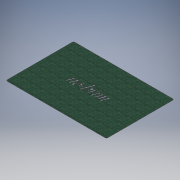
# Autodesk Inventor part: Lamiera logo no-brim
Saved by Autodesk Inventor 2018 (Build 220112000, 112)
## iProperties
Created: 2020-06-01
Part Number: Lamiera logo no-brim
Material: Generico
Document SubType Name: Lamiera
Designer: Francesco
Density: 1 g/cm^3
Sheet Metal Rule: Default_mm
Appearance: Verde - Lucido
Author: Francesco
Autodesk Inventor part; units mm, degrees
ref_plane "YZ Plane" through (0, 0, 0) normal (1, 0, 0) x (0, 1, 0)
ref_plane "XZ Plane" through (0, 0, 0) normal (0, 1, 0) x (-1, 0, 0)
ref_plane "XY Plane" through (0, 0, 0) normal (0, 0, 1) x (1, 0, 0)
sketch "Schizzo1" plane through (0, 0, 0) normal (0, 0, 1) x (1, 0, 0)
  line L0 (-335, 225.25) -> (335, 225.25)
  line L1 (335, 225.25) -> (335, -225.25)
  line L2 (335, -225.25) -> (-335, -225.25)
  line L3 (-335, -225.25) -> (-335, 225.25)
  line L4 (-335, 225.25) -> (335, -225.25) construction
  line L5 (335, 225.25) -> (-335, -225.25) construction
  point P0 (0, 0)
  dimension "d0" = 670
  dimension "d1" = 450.5
  measures "d0" distance of L1.end L2.end
  measures "d1" distance of L0.end L1.end
extrude "Piano1" add sketch "Schizzo1" along normal blind 1
fillet "Arrotondamento angolo1" radius 10 4 edges at (335, 225.25, 0.5) (-335, 225.25, 0.5) (335, -225.25, 0.5) (-335, -225.25, 0.5)
sketch "Schizzo2" plane through (0, 0, 1) normal (0, 0, 1) x (1, 0, 0)
  line L0 (-157.4575, 51.7567) -> (134.7822, 51.7567) construction
  line L1 (134.7822, 51.7567) -> (134.7822, -31.7703) construction
  line L2 (134.7822, -31.7703) -> (-157.4575, -31.7703) construction
  line L3 (-157.4575, -31.7703) -> (-157.4575, 51.7567) construction
  line L4 (-101.4621, -20.1147) -> (-100.5991, -21.6417)
  spline S0 degree 2 poles (-100.5991, -21.6417) (-107.3044, -26.4218) (-116.4663, -28.3471) knots 0 0 0 1 1 1
  spline S1 degree 2 poles (-116.4663, -28.3471) (-115.2713, -19.1189) (-105.5783, -0.3305) knots 0 0 0 1 1 1
  line L5 (-105.5783, -0.3305) -> (-101.9932, 6.5741)
  spline S2 degree 2 poles (-101.9932, 6.5741) (-100.1343, 10.1592) (-100.1343, 11.155) knots 0 0 0 1 1 1
  spline S3 degree 2 poles (-100.1343, 11.155) (-100.1343, 12.682) (-101.3293, 12.682) knots 0 0 0 1 1 1
  spline S4 degree 2 poles (-101.3293, 12.682) (-103.1219, 12.682) (-112.7484, 4.848) (-117.3293, -0.2641) knots 0 0 0 1 2 2 2
  spline S5 degree 2 poles (-117.3293, -0.2641) (-126.8231, -10.8865) (-133.263, -25.7579) knots 0 0 0 1 1 1
  spline S6 degree 2 poles (-133.263, -25.7579) (-135.8522, -26.3554) (-140.6322, -28.4135) knots 0 0 0 1 1 1
  spline S7 degree 2 poles (-140.6322, -28.4135) (-135.5202, -17.9238) (-125.097, 8.2338) (-125.097, 10.6239) knots 0 0 0 1 2 2 2
  spline S8 degree 2 poles (-125.097, 10.6239) (-125.097, 12.6156) (-126.6903, 12.6156) knots 0 0 0 1 1 1
  spline S9 degree 2 poles (-126.6903, 12.6156) (-127.5534, 12.6156) (-130.3418, 11.7525) knots 0 0 0 1 1 1
  spline S10 degree 2 poles (-130.3418, 11.7525) (-130.541, 11.6861) (-130.9393, 11.6197) knots 0 0 0 1 1 1
  line L6 (-130.9393, 11.6197) -> (-131.2713, 13.3459)
  spline S11 degree 2 poles (-131.2713, 13.3459) (-123.4372, 15.6031) (-117.1302, 18.3915) knots 0 0 0 1 1 1
  line L7 (-117.1302, 18.3915) -> (-116.4663, 18.7235)
  spline S12 degree 2 poles (-116.4663, 18.7235) (-116.3335, 17.9932) (-116.3335, 17.7276) knots 0 0 0 1 1 1
  spline S13 degree 2 poles (-116.3335, 17.7276) (-116.3335, 12.7484) (-123.6364, -3.3844) knots 0 0 0 1 1 1
  line L8 (-123.6364, -3.3844) -> (-124.4331, -5.0442)
  line L9 (-124.4331, -5.0442) -> (-123.4372, -3.9819)
  spline S14 degree 2 poles (-123.4372, -3.9819) (-114.3418, 6.4413) (-98.8729, 18.4579) (-94.4912, 18.4579) knots 0 0 0 1 2 2 2
  spline S15 degree 2 poles (-94.4912, 18.4579) (-91.7692, 18.4579) (-91.7692, 15.6695) knots 0 0 0 1 1 1
  spline S16 degree 2 poles (-91.7692, 15.6695) (-91.7692, 12.7484) (-99.0721, -1.4591) knots 0 0 0 1 1 1
  spline S17 degree 2 poles (-99.0721, -1.4591) (-107.8356, -18.4549) (-107.8356, -20.5794) knots 0 0 0 1 1 1
  spline S18 degree 2 poles (-107.8356, -20.5794) (-107.8356, -22.1728) (-106.3086, -22.1728) knots 0 0 0 1 1 1
  spline S19 degree 2 poles (-106.3086, -22.1728) (-104.6488, -22.1728) (-101.7941, -20.3803) knots 0 0 0 1 1 1
  line L10 (-101.7941, -20.3803) -> (-101.4621, -20.1147)
  spline S20 degree 2 poles (-53.7941, 12.9475) (-56.7152, 13.2131) (-58.7069, 13.2131) knots 0 0 0 1 1 1
  spline S21 degree 2 poles (-58.7069, 13.2131) (-73.3791, 13.2131) (-81.2132, 1.9932) knots 0 0 0 1 1 1
  spline S22 degree 2 poles (-81.2132, 1.9932) (-84.2671, -2.5213) (-88.5161, -14.0068) (-88.5161, -17.9238) knots 0 0 0 1 2 2 2
  spline S23 degree 2 poles (-88.5161, -17.9238) (-88.5161, -20.6458) (-85.3293, -24.1645) (-82.8729, -24.1645) knots 0 0 0 1 2 2 2
  spline S24 degree 2 poles (-82.8729, -24.1645) (-77.0306, -24.1645) (-62.9559, -5.5753) (-62.9559, 2.1924) knots 0 0 0 1 2 2 2
  spline S25 degree 2 poles (-62.9559, 2.1924) (-62.9559, 3.9185) (-64.8148, 6.3085) (-66.0762, 6.3085) knots 0 0 0 1 2 2 2
  spline S26 degree 2 poles (-66.0762, 6.3085) (-70.5244, 6.3085) (-74.6405, -2.6541) knots 0 0 0 1 1 1
  spline S27 degree 2 poles (-74.6405, -2.6541) (-74.9061, -1.5255) (-74.9061, -0.6624) knots 0 0 0 1 1 1
  spline S28 degree 2 poles (-74.9061, -0.6624) (-74.9061, 2.7899) (-66.3418, 10.3583) (-62.4248, 10.3583) knots 0 0 0 1 2 2 2
  spline S29 degree 2 poles (-62.4248, 10.3583) (-59.902, 10.3583) (-56.3169, 6.1758) (-56.3169, 3.1882) knots 0 0 0 1 2 2 2
  spline S30 degree 2 poles (-56.3169, 3.1882) (-56.3169, -6.9031) (-69.1966, -18.1894) knots 0 0 0 1 1 1
  spline S31 degree 2 poles (-69.1966, -18.1894) (-80.2837, -28.0151) (-87.5866, -28.0151) knots 0 0 0 1 1 1
  spline S32 degree 2 poles (-87.5866, -28.0151) (-90.7733, -28.0151) (-94.9559, -23.4342) (-94.9559, -19.9819) knots 0 0 0 1 2 2 2
  spline S33 degree 2 poles (-94.9559, -19.9819) (-94.9559, -12.3471) (-84.3335, 4.3168) (-75.57, 10.3583) knots 0 0 0 1 2 2 2
  spline S34 degree 2 poles (-75.57, 10.3583) (-70.7899, 13.6114) (-59.5036, 17.8604) (-55.5202, 17.8604) knots 0 0 0 1 2 2 2
  spline S35 degree 2 poles (-55.5202, 17.8604) (-53.0638, 17.8604) (-53.0638, 15.6695) knots 0 0 0 1 1 1
  spline S36 degree 2 poles (-53.0638, 15.6695) (-53.0638, 14.8065) (-53.7941, 12.9475) knots 0 0 0 1 1 1
  line L11 (-53.9269, -2.2558) -> (-46.292, -2.2558)
  line L12 (-46.292, -2.2558) -> (-44.1011, -2.2558)
  spline S37 degree 2 poles (-44.1011, -2.2558) (-39.653, -2.2558) (-36.6654, -0.7288) knots 0 0 0 1 1 1
  spline S38 degree 2 poles (-36.6654, -0.7288) (-36.5991, -0.6624) (-36.4663, -0.6624) knots 0 0 0 1 1 1
  line L13 (-36.4663, -0.6624) -> (-36.5991, -0.9944)
  line L14 (-36.5991, -0.9944) -> (-36.9974, -1.8574)
  spline S39 degree 2 poles (-36.9974, -1.8574) (-39.2547, -7.0359) (-46.4912, -7.0359) knots 0 0 0 1 1 1
  line L15 (-46.4912, -7.0359) -> (-49.0804, -7.0359)
  line L16 (-49.0804, -7.0359) -> (-51.8688, -7.0359)
  spline S40 degree 2 poles (-51.8688, -7.0359) (-53.8605, -7.0359) (-55.321, -7.7662) (-56.1177, -9.0276) knots 0 0 0 1 2 2 2
  line L17 (-56.1177, -9.0276) -> (-56.4497, -9.5587)
  line L18 (-56.4497, -9.5587) -> (-57.4455, -9.5587)
  line L19 (-57.4455, -9.5587) -> (-53.9269, -2.2558)
  spline S41 degree 2 poles (-6.458, 48.4662) (-7.1219, 40.1011) (-21.7277, 5.3791) knots 0 0 0 1 1 1
  line L20 (-21.7277, 5.3791) -> (-22.7235, 3.1218)
  spline S42 degree 2 poles (-22.7235, 3.1218) (-16.682, 9.6944) (-2.4082, 18.0596) (2.8366, 18.0596) knots 0 0 0 1 2 2 2
  spline S43 degree 2 poles (2.8366, 18.0596) (7.9487, 18.0596) (7.9487, 12.6156) knots 0 0 0 1 1 1
  spline S44 degree 2 poles (7.9487, 12.6156) (7.9487, 6.5077) (-3.2049, -9.8242) (-11.8356, -16.3969) knots 0 0 0 1 2 2 2
  spline S45 degree 2 poles (-11.8356, -16.3969) (-27.57, -28.2143) (-42.2422, -28.2143) knots 0 0 0 1 1 1
  line L21 (-42.2422, -28.2143) -> (-41.5119, -26.4218)
  spline S46 degree 2 poles (-41.5119, -26.4218) (-31.0223, -2.2558) (-15.6862, 36.848) (-15.6862, 39.1716) knots 0 0 0 1 2 2 2
  spline S47 degree 2 poles (-15.6862, 39.1716) (-15.6862, 40.8314) (-17.6779, 40.8314) knots 0 0 0 1 1 1
  spline S48 degree 2 poles (-17.6779, 40.8314) (-18.9393, 40.8314) (-21.6613, 39.8355) knots 0 0 0 1 1 1
  line L22 (-21.6613, 39.8355) -> (-22.3252, 41.5616)
  spline S49 degree 2 poles (-22.3252, 41.5616) (-15.0223, 44.2172) (-6.458, 48.4662) knots 0 0 0 1 1 1
  spline S50 degree 2 poles (-33.8771, -22.6375) (-32.4165, -22.8367) (-31.6198, -22.8367) knots 0 0 0 1 1 1
  spline S51 degree 2 poles (-31.6198, -22.8367) (-19.2713, -22.8367) (-9.5783, -10.4218) knots 0 0 0 1 1 1
  spline S52 degree 2 poles (-9.5783, -10.4218) (-5.6613, -5.3761) (-0.4829, 5.9766) (-0.4829, 9.4953) knots 0 0 0 1 2 2 2
  spline S53 degree 2 poles (-0.4829, 9.4953) (-0.4829, 13.4123) (-4.1343, 13.4123) knots 0 0 0 1 1 1
  spline S54 degree 2 poles (-4.1343, 13.4123) (-10.5078, 13.4123) (-28.4995, -8.4301) (-33.8771, -22.6375) knots 0 0 0 1 2 2 2
  line L23 (41.2765, 17.8604) -> (39.2848, 12.2836)
  spline S55 degree 2 poles (39.2848, 12.2836) (37.1603, 12.7484) (35.5669, 12.7484) knots 0 0 0 1 1 1
  spline S56 degree 2 poles (35.5669, 12.7484) (29.0607, 12.7484) (21.6914, 2.7899) knots 0 0 0 1 1 1
  spline S57 degree 2 poles (21.6914, 2.7899) (18.2391, -1.9238) (13.2599, -13.0774) (9.6084, -24.5628) knots 0 0 0 1 2 2 2
  line L24 (9.6084, -24.5628) -> (9.0109, -26.4218)
  spline S58 degree 2 poles (9.0109, -26.4218) (5.3595, -27.2184) (2.04, -28.3471) knots 0 0 0 1 1 1
  line L25 (2.04, -28.3471) -> (2.7039, -26.6209)
  line L26 (2.7039, -26.6209) -> (7.6167, -13.6085)
  spline S59 degree 2 poles (7.6167, -13.6085) (14.5877, 5.2463) (14.5877, 8.5658) knots 0 0 0 1 1 1
  spline S60 degree 2 poles (14.5877, 8.5658) (14.5877, 10.2919) (13.0607, 10.2919) knots 0 0 0 1 1 1
  spline S61 degree 2 poles (13.0607, 10.2919) (12.264, 10.2919) (9.3429, 8.8314) knots 0 0 0 1 1 1
  line L27 (9.3429, 8.8314) -> (8.6126, 10.5575)
  spline S62 degree 2 poles (8.6126, 10.5575) (16.3802, 14.3417) (22.6209, 18.9226) knots 0 0 0 1 1 1
  spline S63 degree 2 poles (22.6209, 18.9226) (22.82, 17.9268) (22.82, 17.1301) knots 0 0 0 1 1 1
  spline S64 degree 2 poles (22.82, 17.1301) (22.82, 12.8148) (18.9694, 2.7899) knots 0 0 0 1 1 1
  line L28 (18.9694, 2.7899) -> (20.2972, 4.3168)
  spline S65 degree 2 poles (20.2972, 4.3168) (33.3097, 18.6571) (38.6873, 18.6571) knots 0 0 0 1 1 1
  spline S66 degree 2 poles (38.6873, 18.6571) (39.8823, 18.6571) (41.2765, 17.8604) knots 0 0 0 1 1 1
  line L29 (54.0897, 19.4538) -> (54.0897, 18.8563)
  spline S67 degree 2 poles (54.0897, 18.8563) (54.0897, 13.6114) (47.1852, -1.9238) knots 0 0 0 1 1 1
  line L30 (47.1852, -1.9238) -> (43.069, -11.2848)
  spline S68 degree 2 poles (43.069, -11.2848) (39.8159, -18.7869) (39.6831, -20.513) knots 0 0 0 1 1 1
  spline S69 degree 2 poles (39.6831, -20.513) (39.6167, -22.2392) (41.542, -22.1064) knots 0 0 0 1 1 1
  spline S70 degree 2 poles (41.542, -22.1064) (42.6707, -22.04) (45.2599, -20.9114) knots 0 0 0 1 1 1
  line L31 (45.2599, -20.9114) -> (45.9902, -22.5047)
  spline S71 degree 2 poles (45.9902, -22.5047) (37.2267, -26.6873) (31.9819, -28.4798) knots 0 0 0 1 1 1
  spline S72 degree 2 poles (31.9819, -28.4798) (32.2474, -23.235) (35.1022, -14.4052) (39.8159, -4.1147) knots 0 0 0 1 2 2 2
  spline S73 degree 2 poles (39.8159, -4.1147) (45.791, 9.0305) (45.9238, 11.2878) knots 0 0 0 1 1 1
  spline S74 degree 2 poles (45.9238, 11.2878) (46.0565, 13.0139) (44.4632, 13.0139) knots 0 0 0 1 1 1
  spline S75 degree 2 poles (44.4632, 13.0139) (43.7329, 13.0139) (42.6043, 12.6156) knots 0 0 0 1 1 1
  line L32 (42.6043, 12.6156) -> (40.2806, 11.7525)
  spline S76 degree 2 poles (40.2806, 11.7525) (40.0151, 11.6861) (39.2184, 11.3542) knots 0 0 0 1 1 1
  line L33 (39.2184, 11.3542) -> (38.6209, 13.1467)
  line L34 (38.6209, 13.1467) -> (39.8159, 13.5451)
  spline S77 degree 2 poles (39.8159, 13.5451) (45.9902, 15.8023) (52.43, 18.6571) knots 0 0 0 1 1 1
  line L35 (52.43, 18.6571) -> (54.0897, 19.4538)
  spline S78 degree 2 poles (57.3429, 33.7276) (59.9321, 33.7276) (59.9321, 31.1384) knots 0 0 0 1 1 1
  spline S79 degree 2 poles (59.9321, 31.1384) (59.9321, 29.6778) (57.6084, 27.3542) (56.2142, 27.3542) knots 0 0 0 1 2 2 2
  spline S80 degree 2 poles (56.2142, 27.3542) (53.5586, 27.3542) (53.5586, 29.9434) knots 0 0 0 1 1 1
  spline S81 degree 2 poles (53.5586, 29.9434) (53.5586, 31.404) (55.8823, 33.7276) (57.3429, 33.7276) knots 0 0 0 1 2 2 2
  line L36 (107.0026, -19.8491) -> (107.9321, -21.3097)
  spline S82 degree 2 poles (107.9321, -21.3097) (102.0234, -25.5587) (93.8574, -28.2143) knots 0 0 0 1 1 1
  spline S83 degree 2 poles (93.8574, -28.2143) (94.7204, -16.0649) (105.3429, 5.5782) knots 0 0 0 1 1 1
  line L37 (105.3429, 5.5782) -> (106.9362, 9.0305)
  spline S84 degree 2 poles (106.9362, 9.0305) (107.4009, 9.8272) (107.4009, 10.4247) knots 0 0 0 1 1 1
  spline S85 degree 2 poles (107.4009, 10.4247) (107.4009, 11.7525) (106.2059, 11.7525) knots 0 0 0 1 1 1
  spline S86 degree 2 poles (106.2059, 11.7525) (103.8159, 11.7525) (96.7121, 4.6488) knots 0 0 0 1 1 1
  spline S87 degree 2 poles (96.7121, 4.6488) (91.6001, -0.5296) (82.5047, -16.4632) (79.6499, -25.094) knots 0 0 0 1 2 2 2
  spline S88 degree 2 poles (79.6499, -25.094) (76.3304, -25.957) (71.7495, -28.2143) knots 0 0 0 1 1 1
  line L38 (71.7495, -28.2143) -> (72.347, -26.6209)
  line L39 (72.347, -26.6209) -> (75.7329, -18.4549)
  spline S89 degree 2 poles (75.7329, -18.4549) (79.3843, -9.3595) (85.4258, 8.3666) (85.4258, 10.2919) knots 0 0 0 1 2 2 2
  spline S90 degree 2 poles (85.4258, 10.2919) (85.4258, 11.8853) (83.8989, 11.8853) knots 0 0 0 1 1 1
  spline S91 degree 2 poles (83.8989, 11.8853) (82.04, 11.8853) (73.2101, 2.9226) (69.4258, -2.9197) knots 0 0 0 1 2 2 2
  spline S92 degree 2 poles (69.4258, -2.9197) (62.8532, -13.0774) (58.0068, -25.3595) knots 0 0 0 1 1 1
  spline S93 degree 2 poles (58.0068, -25.3595) (57.2765, -25.6251) (57.1437, -25.6251) knots 0 0 0 1 1 1
  line L40 (57.1437, -25.6251) -> (54.1561, -26.6873)
  spline S94 degree 2 poles (54.1561, -26.6873) (52.3636, -27.3512) (50.5047, -28.0815) knots 0 0 0 1 1 1
  spline S95 degree 2 poles (50.5047, -28.0815) (51.8325, -25.2267) (55.7495, -15.7993) knots 0 0 0 1 1 1
  line L41 (55.7495, -15.7993) -> (60.1312, -5.3761)
  spline S96 degree 2 poles (60.1312, -5.3761) (64.9777, 6.5741) (65.1769, 9.5616) knots 0 0 0 1 1 1
  spline S97 degree 2 poles (65.1769, 9.5616) (65.3097, 11.5533) (63.5835, 11.5533) knots 0 0 0 1 1 1
  spline S98 degree 2 poles (63.5835, 11.5533) (62.4549, 11.5533) (60.1976, 10.5575) knots 0 0 0 1 1 1
  line L42 (60.1976, 10.5575) -> (59.5337, 12.35)
  spline S99 degree 2 poles (59.5337, 12.35) (64.3802, 14.209) (72.0151, 18.9226) knots 0 0 0 1 1 1
  line L43 (72.0151, 18.9226) -> (73.2765, 19.7193)
  spline S100 degree 2 poles (73.2765, 19.7193) (73.4092, 18.4579) (73.4092, 17.5948) knots 0 0 0 1 1 1
  spline S101 degree 2 poles (73.4092, 17.5948) (73.4092, 12.8148) (67.6333, -1.2599) knots 0 0 0 1 1 1
  spline S102 degree 2 poles (67.6333, -1.2599) (83.1686, 18.5243) (91.6665, 18.5243) knots 0 0 0 1 1 1
  spline S103 degree 2 poles (91.6665, 18.5243) (94.1893, 18.5243) (94.1893, 15.8687) knots 0 0 0 1 1 1
  spline S104 degree 2 poles (94.1893, 15.8687) (94.1893, 11.8189) (88.5462, -1.9902) knots 0 0 0 1 1 1
  spline S105 degree 2 poles (88.5462, -1.9902) (94.986, 6.4413) (109.9902, 18.5907) (114.04, 18.5907) knots 0 0 0 1 2 2 2
  spline S106 degree 2 poles (114.04, 18.5907) (116.3636, 18.5907) (116.3636, 16.267) knots 0 0 0 1 1 1
  spline S107 degree 2 poles (116.3636, 16.267) (116.3636, 14.6073) (112.1146, 5.5782) knots 0 0 0 1 1 1
  spline S108 degree 2 poles (112.1146, 5.5782) (101.8906, -16.3305) (101.8906, -19.8491) knots 0 0 0 1 1 1
  spline S109 degree 2 poles (101.8906, -19.8491) (101.8906, -21.3761) (103.3512, -21.3761) knots 0 0 0 1 1 1
  spline S110 degree 2 poles (103.3512, -21.3761) (104.4134, -21.3761) (107.0026, -19.8491) knots 0 0 0 1 1 1
  point P0 (0, 0)
  constraints: 2 other
extrude "Estrusione1" cut sketch "Schizzo2" against normal up to next
equation "\"d2\" = Spessore"
equation "\"RaggioPiega\" = Spessore"
equation "\"LarghezzaScaricoPiega\" = Spessore"
equation "\"ProfonditàScaricoPiega\" = 0.5 * Spessore"
equation "\"DimensioniScaricoAngolo\" = 4 * Spessore"
equation "\"ResiduoMinimo\" = 2 * Spessore"
equation "\"RaggioTransizione\" = RaggioPiega"
equation "\"Dimensione_raggio_Jacobi\" = RaggioPiega"
equation "\"DimensioneGioco\" = Spessore"
equation "\"Spessore\" = 1"
